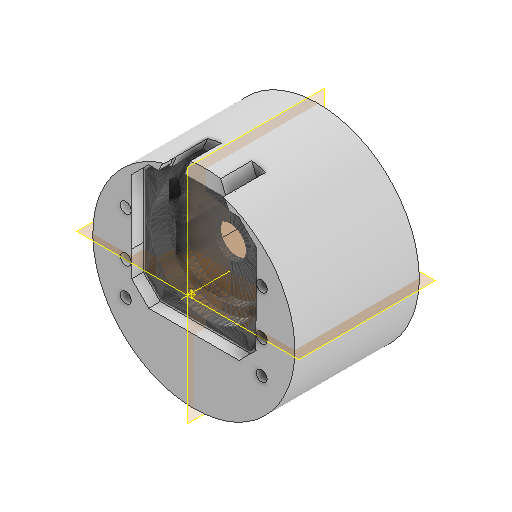
# Autodesk Inventor part: Pump_Base_Motor
Saved by Autodesk Inventor 2022 (Build 260153000, 153)
## iProperties
Created: 2022-11-30
Part Number: Pump_Base_Motor
Material: Generisch
Document SubType Name: Modeling
Designer: diederichbenedict
Density: 1 g/cm^3
Appearance: Vorgabe
Author: diederichbenedict
Autodesk Inventor part; units mm, degrees
note: some values were not read from the file. Chosen so that the rebuilt part matches the saved one: offset side.
ref_plane "XY Plane" through (0, 0, 0) normal (0, 0, 1) x (1, 0, 0)
sketch "Skizze1" plane through (-82.898, -113.257, 0) normal (0, 0, -1) x (-1, 0, 0)
  ellipse E0 centre (-5.6597, 2.5025) end of major axis (-3.7004, 3.2582) minor radius 2.1
  ellipse E1 centre (29.3402, 2.5025) end of major axis (31.2996, 3.2582) minor radius 2.1
  circle A0 centre (-5.6597, 2.5025) radius 1.4
  circle A1 centre (29.3402, 2.5025) radius 1.4
  line L0 (-3.648, 21.791) -> (-3.648, -0.92)
  line L1 (27.352, -0.92) -> (27.352, 21.933)
  ellipse E2 centre (-5.6597, 2.5025) end of major axis (-8.9253, 1.2431) minor radius 3.5 (-5.6597, 6.0025) -> (-5.6598, -0.9974) ccw
  ellipse E3 centre (29.3402, 2.5025) end of major axis (32.6058, 3.762) minor radius 3.5 (32.8402, 2.5025) -> (29.3403, 6.0025) ccw
  ellipse E4 centre (29.3402, 2.5025) end of major axis (32.6058, 3.762) minor radius 3.5 (29.3402, -0.9975) -> (32.8402, 2.5025) ccw
  line L2 (-5.6598, -0.9974) -> (-3.648, -0.92)
  line L3 (-5.6597, 6.0025) -> (-3.648, 6.0025)
  line L4 (29.3403, 6.0025) -> (27.352, 6.0025)
  line L5 (27.352, -0.92) -> (30.0724, -0.9201)
  line L6 (-3.6505, 21.7885) -> (0.568, 26.007)
  line L7 (23.278, 26.007) -> (27.355, 21.932)
  ellipse E5 centre (11.8414, 2.4996) end of major axis (-1.2208, -2.5382) minor radius 13.9999 (20.5913, -8.4291) -> (25.3968, -1.0004) ccw
  line L8 (27.352, -0.92) -> (23.278, -4.993)
  line L9 (0.426, -4.993) -> (-3.648, -0.92)
  line L10 (23.278, 26.007) -> (0.568, 26.007)
  line L11 (-3.6505, 21.7885) -> (-3.648, -0.92)
  line L12 (0.426, -4.993) -> (23.278, -4.993)
  line L13 (27.352, -0.92) -> (27.355, 21.932)
  ellipse E6 centre (11.8519, 3.9724) end of major axis (-12.4064, -5.3836) minor radius 25.9999 (37.8497, 4.307) -> (-0.2097, 27.0053) ccw
  circle A2 centre (11.8519, 3.9724) radius 26
  point P0 (-82.898, 113.257)
  point P1 (27.352, 3.1784)
  point P2 (27.352, 1.8266)
  point P3 (-3.648, 1.9001)
  point P4 (-3.648, 3.105)
  point P5 (-3.6488, 6.0025)
  point P6 (27.3529, 6.0025)
extrude "Extrusion1" add sketch "Skizze1" against normal blind 8 contours E0 L0 | E0 L0 L2 E2 L3 | L1 E1 L4 E3 E4 L5 | L1 E1 | A2 E6 picked at (-3.8519, 2.5026) picked at (27.5482, 2.5026)
sketch "Skizze3" plane through (-94.7499, -109.2846, 0) normal (0, 0, -1) x (-1, 0, 0)
  circle A0 centre (0, 0) radius 26 projected
  line L0 (8.7207, -12.3528) -> (8.7206, -19.924) projected
  line L1 (-8.7794, -19.924) -> (8.7206, -19.924) projected
  line L2 (-8.7794, -19.924) -> (-8.7793, -12.3528) projected
  ellipse E0 centre (-0.032, -1.4169) end of major axis (-13.0942, -6.4548) minor radius 13.9999 projected
  line L3 (-9.2793, -12.3528) -> (-9.2794, -20.424)
  line L4 (-9.2794, -20.424) -> (9.2206, -20.424)
  line L5 (9.2206, -20.424) -> (9.2207, -12.3528)
  line L6 (-13.567, 2.0301) -> (-17.5116, 2.0301) projected
  ellipse E1 centre (-17.5116, -1.4699) end of major axis (-20.7771, -2.7294) minor radius 3.5 (-17.5116, 2.0301) -> (-17.5116, -4.9699) ccw projected
  line L7 (-17.5116, -4.9699) -> (-13.5671, -4.9699) projected
  line L8 (17.4884, 2.03) -> (13.5438, 2.03) projected
  ellipse E2 centre (17.4884, -1.47) end of major axis (20.7539, -0.2105) minor radius 3.5 (20.9884, -1.47) -> (17.4884, 2.03) ccw projected
  ellipse E3 centre (17.4884, -1.47) end of major axis (20.7539, -0.2105) minor radius 3.5 (17.4884, -4.9699) -> (20.9884, -1.47) ccw projected
  line L9 (13.5438, -4.9699) -> (17.4884, -4.9699) projected
  line L10 (13.5438, -5.4699) -> (17.4884, -5.4699)
  line L11 (17.4884, 2.53) -> (13.5438, 2.53)
  line L12 (-13.567, 2.5301) -> (-17.5116, 2.5301)
  line L13 (-17.5116, -5.4699) -> (-13.5671, -5.4699)
  spline S0 degree 5 poles (-13.5607, -6.6347) (-12.2488, -10.0344) (-9.8719, -13.0248) (-6.5899, -15.1472) (0.8113, -17.0371) (7.9664, -14.3613) (11, -11.897) (15.084, -5.4414) (14.7507, 2.1899) (13.3442, 5.8368) (8.4668, 11.7155) (1.1057, 13.7569) (-2.797, 13.546) (-9.8958, 10.7242) (-14.1112, 4.3539) (-15.118, 0.5774) (-14.8714, -3.2345) (-13.5607, -6.6347) knots 0 0 0 0 0 0 0.2 0.2 0.2 0.4 0.4 0.4 0.6 0.6 0.6 0.8 0.8 0.8 1 1 1 1 1 1
  spline S1 degree 5 poles (17.4884, -5.4699) (18.1167, -5.47) (18.745, -5.3466) (19.341, -5.0998) (20.404, -4.3856) (21.1182, -3.3226) (21.365, -2.7266) (21.4884, -2.0983) (21.4884, -1.47) knots 0 0 0 0 0 0 0.5 0.5 0.5 1 1 1 1 1 1
  spline S2 degree 5 poles (21.4884, -1.47) (21.4884, -0.8416) (21.365, -0.2133) (21.1182, 0.3827) (20.404, 1.4456) (19.341, 2.1599) (18.745, 2.4066) (18.1167, 2.53) (17.4884, 2.53) knots 0 0 0 0 0 0 0.5 0.5 0.5 1 1 1 1 1 1
  spline S3 degree 5 poles (-17.5116, 2.5301) (-18.2237, 2.5301) (-18.9358, 2.3715) (-19.6009, 2.0547) (-21.0453, 0.9066) (-21.7037, -0.8783) (-21.7037, -2.0614) (-21.0453, -3.8464) (-19.6009, -4.9945) (-18.9358, -5.3113) (-18.2237, -5.4699) (-17.5116, -5.4699) knots 0 0 0 0 0 0 0.283333 0.283333 0.283333 0.716667 0.716667 0.716667 1 1 1 1 1 1
  point P0 (-94.7499, 109.2846)
  point P1 (-9.2793, -12.5855)
  point P2 (9.2207, -12.581)
  point P3 (13.89, -5.4699)
  point P4 (13.9204, 2.53)
  point P5 (-13.9845, 2.5301)
  point P6 (-13.9541, -5.4699)
  dimension "d4" = 0.5
  dimension "d5" = 0.5
  dimension "d6" = 0.5
  dimension "d7" = 0.5
  constraints: 14 end point, 6 point on line, 4 parallel, 22 other
  measures "d5" distance between parallel lines of L2 L3
  measures "d6" distance between parallel lines of L9 L10
  measures "d7" distance between parallel lines of L6 L12
ref_plane "Arbeitsebene1" through (-103.4705, -129.2086, -18.5626) normal (-0.001105, -0.0028651, 0.9999953) x (0.9999994, 0.0000016, 0.001105)
extrude "Extrusion2" add sketch "Skizze3" along normal blind 21
sketch "Skizze4" plane through (-94.7499, -109.2846, 8) normal (0, 0, 1) x (1, 0, 0)
  line L0 (-5.4471, 22.0346) -> (-6.7391, 18.9176) projected
  line L1 (-8.6961, 22.0346) -> (-12.197, 13.5825) projected
  line L2 (-15.5031, 17.9596) -> (-15.5011, 2.53) projected
  line L3 (-13.9205, 2.53) -> (-15.5011, 2.53) projected
  line L4 (15.5007, 2.5301) -> (13.9845, 2.5301) projected
  line L5 (15.5007, 2.5301) -> (15.5024, 17.8161) projected
  line L6 (15.5024, 17.8161) -> (11.2839, 22.0346) projected
  line L7 (11.2839, 22.0346) -> (-11.4261, 22.0346) projected
  line L8 (-11.4261, 22.0346) -> (-15.5031, 17.9596) projected
  line L9 (5.4339, 22.0346) -> (6.7219, 18.9276) projected
  line L10 (8.6829, 22.0346) -> (12.1573, 13.6483) projected
  line L11 (-8.6961, 22.0346) -> (-6.7659, 26.6912)
  line L12 (-6.7659, 26.6912) -> (-3.291, 27.2362)
  line L13 (-3.291, 27.2362) -> (-5.4471, 22.0346)
  line L14 (-8.6961, 22.0346) -> (-5.4471, 22.0346)
  line L15 (11.2839, 22.0346) -> (-11.4261, 22.0346) projected
  line L16 (5.4339, 22.0346) -> (3.2998, 27.1825)
  line L17 (3.2998, 27.1825) -> (6.55, 27.1825)
  line L18 (6.55, 27.1825) -> (8.6829, 22.0346)
  point P0 (94.7499, 109.2846)
  constraints: 14 end point, 4 collinear, 2 parallel, 1 other
extrude "Extrusion3" cut sketch "Skizze4" against normal up to surface (8 mm away)
sketch "Skizze5" plane through (-94.7499, -109.2846, -21) normal (0, 0, -1) x (-0.9330107, 0.3598486, 0)
  line L0 (7.393, -19.5794) -> (14.0269, -2.3795) projected
  line L1 (9.2521, -0.5379) -> (2.6182, -17.7379) projected
  line L2 (-13.4636, -11.5246) -> (-6.8359, 5.6595) projected
  line L3 (-11.6237, 7.5061) -> (-18.2515, -9.678) projected
  ellipse E0 centre (-7.4951, -21.5592) end of major axis (-4.3201, -21.5592) minor radius 3.175 (-8.5377, -24.5581) -> (-4.5153, -22.6553) ccw projected
  ellipse E1 centre (0, 0) end of major axis (-26, 0) minor radius 25.9999 (-16.1994, 20.3365) -> (-8.5377, -24.5581) ccw projected
  ellipse E2 centre (-14.2212, 17.8531) end of major axis (-17.3962, 17.8531) minor radius 3.175 (-11.5991, 19.6434) -> (-16.1994, 20.3365) ccw projected
  ellipse E3 centre (-8.915, 21.476) end of major axis (-5.665, 21.476) minor radius 3.25 (-11.5991, 19.6434) -> (-5.7222, 22.083) ccw projected
  ellipse E4 centre (-2.6031, 22.676) end of major axis (-5.7781, 22.676) minor radius 3.175 (-2.9652, 25.8302) -> (-5.7222, 22.083) ccw projected
  ellipse E5 centre (0, 0) end of major axis (-26, 0) minor radius 25.9999 (24.3766, -9.0431) -> (-2.9652, 25.8302) ccw projected
  ellipse E6 centre (21.3999, -7.9388) end of major axis (24.5749, -7.9388) minor radius 3.175 (20.3498, -10.9351) -> (24.3766, -9.0431) ccw projected
  ellipse E7 centre (19.2749, -14.0022) end of major axis (22.5249, -14.0022) minor radius 3.25 (20.3498, -10.9351) -> (16.6903, -15.9726) ccw projected
  ellipse E8 centre (14.1653, -17.8975) end of major axis (17.3403, -17.8975) minor radius 3.175 (16.1358, -20.3871) -> (16.6903, -15.9726) ccw projected
  ellipse E9 centre (0, 0) end of major axis (-26, 0) minor radius 25.9999 (5.4581, -25.4205) -> (16.1358, -20.3871) ccw projected
  ellipse E10 centre (4.7916, -22.3163) end of major axis (7.9666, -22.3163) minor radius 3.175 (1.6998, -23.0382) -> (5.4581, -25.4205) ccw projected
  ellipse E11 centre (-1.4651, -23.7773) end of major axis (1.7849, -23.7773) minor radius 3.25 (1.6998, -23.0382) -> (-4.5153, -22.6553) ccw projected
  ellipse E12 centre (11.6395, -1.4587) end of major axis (9.0807, -1.4587) minor radius 2.5588 (14.0269, -2.3795) -> (9.2521, -0.5379) ccw projected
  ellipse E13 centre (5.0056, -18.6586) end of major axis (7.5644, -18.6586) minor radius 2.5588 (2.6182, -17.7379) -> (7.393, -19.5794) ccw projected
  ellipse E14 centre (-9.2298, 6.5828) end of major axis (-11.7956, 6.5828) minor radius 2.5658 (-6.8359, 5.6595) -> (-11.6237, 7.5061) ccw projected
  ellipse E15 centre (-15.8575, -10.6013) end of major axis (-13.2917, -10.6013) minor radius 2.5658 (-18.2515, -9.678) -> (-13.4636, -11.5246) ccw projected
  ellipse E16 centre (12.7292, -15.6274) end of major axis (15.9792, -15.6274) minor radius 3.25 projected
  ellipse E17 centre (-12.7292, 15.6274) end of major axis (-9.4792, 15.6274) minor radius 3.25 projected
  ellipse E18 centre (-19.9262, -3.0327) end of major axis (-16.6762, -3.0327) minor radius 3.25 projected
  ellipse E19 centre (19.9262, 3.0327) end of major axis (23.1762, 3.0327) minor radius 3.25 projected
  point P0 (-49.0767, 136.0593)
  constraints: 16 other
hole "Bohrung1" at (-112.2499, -99.2846, -21) at (-112.2498, -119.2846, -21) at (-77.2499, -99.2846, -21) at (-77.2498, -119.2845, -21) direction (0, 0, 1) diameter 2.8 end through all counterbore diameter 6.5 counterbore depth 23
sketch "Skizze7" plane through (-82.898, -113.257, 8) normal (0, 0, 1) x (1, 0, 0)
  arc A0 (-19.3639, 28.8636) -> (-4.3543, 28.868) centre (-11.8519, 3.9724) ccw projected
  line L0 (-0.44, -5.0734) -> (3.6345, -0.9829) projected
  line L1 (-4.3543, 28.868) -> (-3.169, 26.007) projected
  line L2 (-3.169, 26.007) -> (-0.568, 26.007) projected
  line L3 (-0.568, 26.007) -> (3.6505, 21.7885) projected
  line L4 (3.6505, 21.7885) -> (3.6488, 6.0025) projected
  line L5 (3.6488, 6.0025) -> (3.648, 6.0025) projected
  line L6 (3.648, 6.0025) -> (3.648, -0.92) projected
  line L7 (3.648, -0.92) -> (-0.426, -4.993) projected
  line L8 (-0.426, -4.993) -> (-23.278, -4.993) projected
  line L9 (-23.278, -4.993) -> (-27.352, -0.92) projected
  line L10 (-27.352, -0.92) -> (-27.352, 6.0025) projected
  line L11 (-27.352, 6.0025) -> (-27.3529, 6.0025) projected
  line L12 (-27.3529, 6.0025) -> (-27.355, 21.932) projected
  line L13 (-27.355, 21.932) -> (-23.278, 26.007) projected
  line L14 (-23.278, 26.007) -> (-20.548, 26.007) projected
  line L15 (-20.548, 26.007) -> (-19.3639, 28.8636) projected
  arc A1 (-19.3639, 28.8636) -> (-4.3543, 28.868) centre (-11.8519, 3.9724) ccw projected
  circle A2 centre (-29.3402, 2.5025) radius 1.4 projected
  circle A3 centre (5.6597, 2.5025) radius 1.4 projected
  line L16 (-0.9329, 25.7138) -> (3.137, 21.6257)
  line L17 (3.137, 21.6257) -> (3.1345, -0.7763)
  line L18 (3.1345, -0.7763) -> (-0.7942, -4.7206)
  line L19 (-23.4851, -5.493) -> (-0.2189, -5.493)
  line L20 (-0.2189, -5.493) -> (4.148, -1.1271)
  line L21 (4.148, -1.1271) -> (4.148, 5.5025)
  line L22 (4.148, 5.5025) -> (4.1487, 5.5025)
  line L23 (4.1487, 5.5025) -> (4.1505, 21.9956)
  line L24 (4.1505, 21.9956) -> (-0.3609, 26.507)
  line L25 (-0.3609, 26.507) -> (-2.8349, 26.507)
  line L26 (-2.8349, 26.507) -> (-3.4776, 28.0582)
  arc A4 (-20.2412, 28.0529) -> (-3.4776, 28.0582) centre (-11.8519, 3.9724) ccw
  line L27 (-20.2412, 28.0529) -> (-20.882, 26.507)
  line L28 (-20.882, 26.507) -> (-23.485, 26.507)
  line L29 (-23.485, 26.507) -> (-27.855, 22.1392)
  line L30 (-27.855, 22.1392) -> (-27.8528, 5.5025)
  line L31 (-27.8528, 5.5025) -> (-27.852, 5.5025)
  line L32 (-27.852, 5.5025) -> (-27.852, -1.1271)
  line L33 (-27.852, -1.1271) -> (-23.4851, -5.493)
  line L34 (-3.4776, 28.0582) -> (-4.3543, 28.868)
  line L35 (-19.3639, 28.8636) -> (-20.548, 26.007) projected
  line L36 (-20.2412, 28.0529) -> (-19.3639, 28.8636)
  circle A5 centre (5.6597, 2.5025) radius 1.4 projected
  circle A6 centre (5.6481, 13.9724) radius 1.4 projected
  circle A7 centre (-29.3519, 13.9724) radius 1.4 projected
  circle A8 centre (-29.3402, 2.5025) radius 1.4 projected
  circle A9 centre (5.6482, -6.0275) radius 1.4 projected
  circle A10 centre (-29.3518, -6.0275) radius 1.4 projected
  point P0 (82.898, 113.257)
  dimension "d22" = 0.5
  constraints: 40 end point, 2 point on circle, 1 centre point, 15 other
  measures "d22" distance between parallel lines of L8 L19
extrude "Extrusion5" add sketch "Skizze7" along normal blind 3 contours L36 A4 L34 A0 | L27 L28 L29 L30 L32 L33 L19 L20 L21 L23 L24 L25 L26 A4
ref_plane "Arbeitsebene2" through (-94.7499, -109.2846, 11) normal (1, 0, 0) x (0, 1, 0)
ref_plane "Arbeitsebene3" through (-94.7499, -109.2846, 11) normal (0, 1, 0) x (-1, 0, 0)
